Autodesk Inventor part; units mm, degrees
(part 2 of 2)
  line L280 (-42.5388, -23.0761) -> (-41.4675, -19.9061)
  line L281 (-41.4675, -19.9061) -> (-40.5993, -19.9061)
  line L282 (-40.5993, -19.9061) -> (-39.528, -23.0761)
  line L283 (-39.528, -23.0761) -> (-40.3475, -23.0761)
  line L284 (-40.3475, -23.0761) -> (-40.5453, -22.4288)
  line L285 (-40.5453, -22.4288) -> (-41.542, -22.4288)
  line L286 (-41.542, -22.4288) -> (-41.7424, -23.0761)
  line L287 (-41.7424, -23.0761) -> (-42.5388, -23.0761)
  line L288 (-40.72, -21.8533) -> (-41.0437, -20.8052)
  line L289 (-41.0437, -20.8052) -> (-41.3699, -21.8533)
  line L290 (-41.3699, -21.8533) -> (-40.72, -21.8533)
  line L291 (-36.4968, -23.0761) -> (-37.2623, -23.0761)
  line L292 (-37.2623, -23.0761) -> (-38.4851, -20.8669)
  line L293 (-38.4851, -20.8669) -> (-38.4851, -23.0761)
  line L294 (-38.4851, -23.0761) -> (-39.2121, -23.0761)
  line L295 (-39.2121, -23.0761) -> (-39.2121, -19.9061)
  line L296 (-39.2121, -19.9061) -> (-38.2359, -19.9061)
  line L297 (-38.2359, -19.9061) -> (-37.2237, -21.7223)
  line L298 (-37.2237, -21.7223) -> (-37.2237, -19.9061)
  line L299 (-37.2237, -19.9061) -> (-36.4968, -19.9061)
  line L300 (-36.4968, -19.9061) -> (-36.4968, -23.0761)
  line L301 (-50.6873, -28.2954) -> (-50.6873, -25.7291)
  line L302 (-50.6873, -25.7291) -> (-51.6249, -25.7291)
  line L303 (-51.6249, -25.7291) -> (-51.6249, -25.1254)
  line L304 (-51.6249, -25.1254) -> (-48.9533, -25.1254)
  line L305 (-48.9533, -25.1254) -> (-48.9533, -25.7291)
  line L306 (-48.9533, -25.7291) -> (-49.8909, -25.7291)
  line L307 (-49.8909, -25.7291) -> (-49.8909, -28.2954)
  line L308 (-49.8909, -28.2954) -> (-50.6873, -28.2954)
  line L309 (-48.9687, -28.2954) -> (-47.8974, -25.1254)
  line L310 (-47.8974, -25.1254) -> (-47.0292, -25.1254)
  line L311 (-47.0292, -25.1254) -> (-45.9579, -28.2954)
  line L312 (-45.9579, -28.2954) -> (-46.7774, -28.2954)
  line L313 (-46.7774, -28.2954) -> (-46.9752, -27.6481)
  line L314 (-46.9752, -27.6481) -> (-47.9719, -27.6481)
  line L315 (-47.9719, -27.6481) -> (-48.1723, -28.2954)
  line L316 (-48.1723, -28.2954) -> (-48.9687, -28.2954)
  line L317 (-47.1499, -27.0727) -> (-47.4736, -26.0246)
  line L318 (-47.4736, -26.0246) -> (-47.7998, -27.0727)
  line L319 (-47.7998, -27.0727) -> (-47.1499, -27.0727)
  line L320 (-42.7134, -28.2954) -> (-43.6819, -28.2954)
  line L321 (-43.6819, -28.2954) -> (-44.563, -27.1317)
  line L322 (-44.563, -27.1317) -> (-44.8508, -27.1317)
  line L323 (-44.8508, -27.1317) -> (-44.8508, -28.2954)
  line L324 (-44.8508, -28.2954) -> (-45.642, -28.2954)
  line L325 (-45.642, -28.2954) -> (-45.642, -25.1254)
  line L326 (-45.642, -25.1254) -> (-44.3678, -25.1254)
  spline S229 degree 2 poles (-44.3678, -25.1254) (-44.1032, -25.1254) (-43.7127, -25.1922) (-43.5458, -25.295) knots 0 0 0 1 2 2 2
  spline S230 degree 2 poles (-43.5458, -25.295) (-43.3762, -25.4029) (-43.1758, -25.7394) (-43.1758, -25.9963) knots 0 0 0 1 2 2 2
  spline S231 degree 2 poles (-43.1758, -25.9963) (-43.1758, -26.3585) (-43.5047, -26.8132) (-43.7795, -26.9468) knots 0 0 0 1 2 2 2
  line L327 (-43.7795, -26.9468) -> (-42.7134, -28.2954)
  spline S232 degree 2 poles (-43.9927, -26.0965) (-43.9927, -25.9757) (-44.0852, -25.8036) (-44.1906, -25.7574) knots 0 0 0 1 2 2 2
  spline S233 degree 2 poles (-44.1906, -25.7574) (-44.265, -25.7266) (-44.4474, -25.7086) (-44.5836, -25.7086) knots 0 0 0 1 2 2 2
  line L328 (-44.5836, -25.7086) -> (-44.8508, -25.7086)
  line L329 (-44.8508, -25.7086) -> (-44.8508, -26.5615)
  line L330 (-44.8508, -26.5615) -> (-44.6221, -26.5615)
  spline S234 degree 2 poles (-44.6221, -26.5615) (-44.4577, -26.5615) (-44.2239, -26.5203) (-44.1443, -26.4561) knots 0 0 0 1 2 2 2
  spline S235 degree 2 poles (-44.1443, -26.4561) (-44.0672, -26.3945) (-43.9927, -26.2301) (-43.9927, -26.0965) knots 0 0 0 1 2 2 2
  line L331 (-39.8312, -25.1254) -> (-40.9204, -28.2954)
  line L332 (-40.9204, -28.2954) -> (-41.7501, -28.2954)
  line L333 (-41.7501, -28.2954) -> (-42.8393, -25.1254)
  line L334 (-42.8393, -25.1254) -> (-42.0147, -25.1254)
  line L335 (-42.0147, -25.1254) -> (-41.3237, -27.2756)
  line L336 (-41.3237, -27.2756) -> (-40.6352, -25.1254)
  line L337 (-40.6352, -25.1254) -> (-39.8312, -25.1254)
  line L338 (-37.9584, -28.2954) -> (-39.6642, -28.2954)
  line L339 (-39.6642, -28.2954) -> (-39.6642, -27.7431)
  line L340 (-39.6642, -27.7431) -> (-39.2095, -27.7431)
  line L341 (-39.2095, -27.7431) -> (-39.2095, -25.6778)
  line L342 (-39.2095, -25.6778) -> (-39.6642, -25.6778)
  line L343 (-39.6642, -25.6778) -> (-39.6642, -25.1254)
  line L344 (-39.6642, -25.1254) -> (-37.9584, -25.1254)
  line L345 (-37.9584, -25.1254) -> (-37.9584, -25.6778)
  line L346 (-37.9584, -25.6778) -> (-38.4131, -25.6778)
  line L347 (-38.4131, -25.6778) -> (-38.4131, -27.7431)
  line L348 (-38.4131, -27.7431) -> (-37.9584, -27.7431)
  line L349 (-37.9584, -27.7431) -> (-37.9584, -28.2954)
  line L350 (-36.8204, -28.2954) -> (-36.8204, -25.7291)
  line L351 (-36.8204, -25.7291) -> (-37.7581, -25.7291)
  line L352 (-37.7581, -25.7291) -> (-37.7581, -25.1254)
  line L353 (-37.7581, -25.1254) -> (-35.0864, -25.1254)
  line L354 (-35.0864, -25.1254) -> (-35.0864, -25.7291)
  line L355 (-35.0864, -25.7291) -> (-36.0241, -25.7291)
  line L356 (-36.0241, -25.7291) -> (-36.0241, -28.2954)
  line L357 (-36.0241, -28.2954) -> (-36.8204, -28.2954)
  spline S236 degree 2 poles (-47.7587, -32.1199) (-47.7587, -32.8828) (-48.8377, -33.9618) (-49.6006, -33.9618) knots 0 0 0 1 2 2 2
  spline S237 degree 2 poles (-49.6006, -33.9618) (-50.3636, -33.9618) (-51.4425, -32.8828) (-51.4425, -32.1199) knots 0 0 0 1 2 2 2
  spline S238 degree 2 poles (-51.4425, -32.1199) (-51.4425, -31.3569) (-50.3636, -30.278) (-49.6006, -30.278) knots 0 0 0 1 2 2 2
  spline S239 degree 2 poles (-49.6006, -30.278) (-48.8377, -30.278) (-47.7587, -31.3569) (-47.7587, -32.1199) knots 0 0 0 1 2 2 2
  spline S240 degree 2 poles (-48.1646, -32.1199) (-48.1646, -31.5265) (-49.0072, -30.6736) (-49.6006, -30.6736) knots 0 0 0 1 2 2 2
  spline S241 degree 2 poles (-49.6006, -30.6736) (-50.194, -30.6736) (-51.0366, -31.5265) (-51.0366, -32.1199) knots 0 0 0 1 2 2 2
  spline S242 degree 2 poles (-51.0366, -32.1199) (-51.0366, -32.7133) (-50.194, -33.5661) (-49.6006, -33.5661) knots 0 0 0 1 2 2 2
  spline S243 degree 2 poles (-49.6006, -33.5661) (-49.0072, -33.5661) (-48.1646, -32.7133) (-48.1646, -32.1199) knots 0 0 0 1 2 2 2
  spline S244 degree 2 poles (-48.925, -32.9239) (-48.9815, -32.9496) (-49.1023, -33.0036) (-49.187, -33.0267) knots 0 0 0 1 2 2 2
  spline S245 degree 2 poles (-49.187, -33.0267) (-49.2744, -33.0524) (-49.4105, -33.0781) (-49.5158, -33.0781) knots 0 0 0 1 2 2 2
  spline S246 degree 2 poles (-49.5158, -33.0781) (-49.7136, -33.0781) (-50.0707, -32.9599) (-50.2017, -32.8392) knots 0 0 0 1 2 2 2
  spline S247 degree 2 poles (-50.2017, -32.8392) (-50.3353, -32.7158) (-50.4894, -32.3588) (-50.4894, -32.1096) knots 0 0 0 1 2 2 2
  spline S248 degree 2 poles (-50.4894, -32.1096) (-50.4894, -31.8733) (-50.3379, -31.5136) (-50.2043, -31.3877) knots 0 0 0 1 2 2 2
  spline S249 degree 2 poles (-50.2043, -31.3877) (-50.0733, -31.2644) (-49.7136, -31.1334) (-49.5158, -31.1334) knots 0 0 0 1 2 2 2
  spline S250 degree 2 poles (-49.5158, -31.1334) (-49.354, -31.1334) (-49.0534, -31.2208) (-48.925, -31.285) knots 0 0 0 1 2 2 2
  line L358 (-48.925, -31.285) -> (-48.925, -31.7191)
  line L359 (-48.925, -31.7191) -> (-48.9687, -31.7191)
  spline S251 degree 2 poles (-48.9687, -31.7191) (-49.0098, -31.6883) (-49.1048, -31.6215) (-49.1819, -31.583) knots 0 0 0 1 2 2 2
  spline S252 degree 2 poles (-49.1819, -31.583) (-49.2487, -31.5496) (-49.4182, -31.5033) (-49.5056, -31.5033) knots 0 0 0 1 2 2 2
  spline S253 degree 2 poles (-49.5056, -31.5033) (-49.7316, -31.5033) (-49.9757, -31.8116) (-49.9757, -32.1096) knots 0 0 0 1 2 2 2
  spline S254 degree 2 poles (-49.9757, -32.1096) (-49.9757, -32.3999) (-49.7265, -32.7081) (-49.5056, -32.7081) knots 0 0 0 1 2 2 2
  spline S255 degree 2 poles (-49.5056, -32.7081) (-49.4079, -32.7081) (-49.2333, -32.6593) (-49.1716, -32.6259) knots 0 0 0 1 2 2 2
  spline S256 degree 2 poles (-49.1716, -32.6259) (-49.0997, -32.5874) (-49.0021, -32.5206) (-48.9687, -32.4924) knots 0 0 0 1 2 2 2
  line L360 (-48.9687, -32.4924) -> (-48.925, -32.4924)
  line L361 (-48.925, -32.4924) -> (-48.925, -32.9239)
  spline S257 degree 2 poles (-43.7102, -32.1199) (-43.7102, -32.8828) (-44.7891, -33.9618) (-45.5521, -33.9618) knots 0 0 0 1 2 2 2
  spline S258 degree 2 poles (-45.5521, -33.9618) (-46.315, -33.9618) (-47.3939, -32.8828) (-47.3939, -32.1199) knots 0 0 0 1 2 2 2
  spline S259 degree 2 poles (-47.3939, -32.1199) (-47.3939, -31.3569) (-46.315, -30.278) (-45.5521, -30.278) knots 0 0 0 1 2 2 2
  spline S260 degree 2 poles (-45.5521, -30.278) (-44.7891, -30.278) (-43.7102, -31.3569) (-43.7102, -32.1199) knots 0 0 0 1 2 2 2
  spline S261 degree 2 poles (-44.1161, -32.1199) (-44.1161, -31.5265) (-44.9586, -30.6736) (-45.5521, -30.6736) knots 0 0 0 1 2 2 2
  spline S262 degree 2 poles (-45.5521, -30.6736) (-46.1455, -30.6736) (-46.9881, -31.5265) (-46.9881, -32.1199) knots 0 0 0 1 2 2 2
  spline S263 degree 2 poles (-46.9881, -32.1199) (-46.9881, -32.7133) (-46.1455, -33.5661) (-45.5521, -33.5661) knots 0 0 0 1 2 2 2
  spline S264 degree 2 poles (-45.5521, -33.5661) (-44.9586, -33.5661) (-44.1161, -32.7133) (-44.1161, -32.1199) knots 0 0 0 1 2 2 2
  spline S265 degree 2 poles (-44.8764, -32.9239) (-44.933, -32.9496) (-45.0537, -33.0036) (-45.1385, -33.0267) knots 0 0 0 1 2 2 2
  spline S266 degree 2 poles (-45.1385, -33.0267) (-45.2258, -33.0524) (-45.362, -33.0781) (-45.4673, -33.0781) knots 0 0 0 1 2 2 2
  spline S267 degree 2 poles (-45.4673, -33.0781) (-45.6651, -33.0781) (-46.0222, -32.9599) (-46.1532, -32.8392) knots 0 0 0 1 2 2 2
  spline S268 degree 2 poles (-46.1532, -32.8392) (-46.2868, -32.7158) (-46.4409, -32.3588) (-46.4409, -32.1096) knots 0 0 0 1 2 2 2
  spline S269 degree 2 poles (-46.4409, -32.1096) (-46.4409, -31.8733) (-46.2893, -31.5136) (-46.1557, -31.3877) knots 0 0 0 1 2 2 2
  spline S270 degree 2 poles (-46.1557, -31.3877) (-46.0247, -31.2644) (-45.6651, -31.1334) (-45.4673, -31.1334) knots 0 0 0 1 2 2 2
  spline S271 degree 2 poles (-45.4673, -31.1334) (-45.3054, -31.1334) (-45.0049, -31.2208) (-44.8764, -31.285) knots 0 0 0 1 2 2 2
  line L362 (-44.8764, -31.285) -> (-44.8764, -31.7191)
  line L363 (-44.8764, -31.7191) -> (-44.9201, -31.7191)
  spline S272 degree 2 poles (-44.9201, -31.7191) (-44.9612, -31.6883) (-45.0563, -31.6215) (-45.1333, -31.583) knots 0 0 0 1 2 2 2
  spline S273 degree 2 poles (-45.1333, -31.583) (-45.2001, -31.5496) (-45.3697, -31.5033) (-45.457, -31.5033) knots 0 0 0 1 2 2 2
  spline S274 degree 2 poles (-45.457, -31.5033) (-45.6831, -31.5033) (-45.9271, -31.8116) (-45.9271, -32.1096) knots 0 0 0 1 2 2 2
  spline S275 degree 2 poles (-45.9271, -32.1096) (-45.9271, -32.3999) (-45.6779, -32.7081) (-45.457, -32.7081) knots 0 0 0 1 2 2 2
  spline S276 degree 2 poles (-45.457, -32.7081) (-45.3594, -32.7081) (-45.1847, -32.6593) (-45.1231, -32.6259) knots 0 0 0 1 2 2 2
  spline S277 degree 2 poles (-45.1231, -32.6259) (-45.0511, -32.5874) (-44.9535, -32.5206) (-44.9201, -32.4924) knots 0 0 0 1 2 2 2
  line L364 (-44.9201, -32.4924) -> (-44.8764, -32.4924)
  line L365 (-44.8764, -32.4924) -> (-44.8764, -32.9239)
  line L366 (-48.9738, -38.7341) -> (-51.3038, -38.7341)
  line L367 (-51.3038, -38.7341) -> (-51.3038, -38.2177)
  spline S278 degree 2 poles (-51.3038, -38.2177) (-51.0084, -37.9814) (-50.5357, -37.5652) (-50.3584, -37.3777) knots 0 0 0 1 2 2 2
  spline S279 degree 2 poles (-50.3584, -37.3777) (-50.1247, -37.1337) (-49.9166, -36.7612) (-49.9166, -36.566) knots 0 0 0 1 2 2 2
  spline S280 degree 2 poles (-49.9166, -36.566) (-49.9166, -36.345) (-50.1812, -36.1087) (-50.4175, -36.1087) knots 0 0 0 1 2 2 2
  spline S281 degree 2 poles (-50.4175, -36.1087) (-50.5383, -36.1087) (-50.754, -36.1678) (-50.8645, -36.214) knots 0 0 0 1 2 2 2
  spline S282 degree 2 poles (-50.8645, -36.214) (-50.9724, -36.2628) (-51.1265, -36.3656) (-51.1651, -36.3913) knots 0 0 0 1 2 2 2
  line L368 (-51.1651, -36.3913) -> (-51.2267, -36.3913)
  line L369 (-51.2267, -36.3913) -> (-51.2267, -35.7002)
  spline S283 degree 2 poles (-51.2267, -35.7002) (-51.0931, -35.636) (-50.5228, -35.5024) (-50.2582, -35.5024) knots 0 0 0 1 2 2 2
  spline S284 degree 2 poles (-50.2582, -35.5024) (-49.6931, -35.5024) (-49.1125, -36.0059) (-49.1125, -36.4606) knots 0 0 0 1 2 2 2
  spline S285 degree 2 poles (-49.1125, -36.4606) (-49.1125, -36.7406) (-49.3771, -37.2801) (-49.6828, -37.5884) knots 0 0 0 1 2 2 2
  spline S286 degree 2 poles (-49.6828, -37.5884) (-49.8755, -37.7785) (-50.2377, -38.0739) (-50.3173, -38.1355) knots 0 0 0 1 2 2 2
  line L370 (-50.3173, -38.1355) -> (-48.9738, -38.1355)
  line L371 (-48.9738, -38.1355) -> (-48.9738, -38.7341)
  spline S287 degree 2 poles (-46.2379, -37.1491) (-46.2379, -37.5601) (-46.369, -38.1766) (-46.5154, -38.3847) knots 0 0 0 1 2 2 2
  spline S288 degree 2 poles (-46.5154, -38.3847) (-46.6592, -38.5902) (-47.1242, -38.8009) (-47.4582, -38.8009) knots 0 0 0 1 2 2 2
  spline S289 degree 2 poles (-47.4582, -38.8009) (-47.7947, -38.8009) (-48.2571, -38.5902) (-48.4035, -38.3796) knots 0 0 0 1 2 2 2
  spline S290 degree 2 poles (-48.4035, -38.3796) (-48.5499, -38.1715) (-48.681, -37.5601) (-48.681, -37.1491) knots 0 0 0 1 2 2 2
  spline S291 degree 2 poles (-48.681, -37.1491) (-48.681, -36.7278) (-48.5499, -36.1318) (-48.4009, -35.916) knots 0 0 0 1 2 2 2
  spline S292 degree 2 poles (-48.4009, -35.916) (-48.252, -35.7054) (-47.7818, -35.4999) (-47.4582, -35.4999) knots 0 0 0 1 2 2 2
  spline S293 degree 2 poles (-47.4582, -35.4999) (-47.1165, -35.4999) (-46.6592, -35.7157) (-46.5128, -35.9289) knots 0 0 0 1 2 2 2
  spline S294 degree 2 poles (-46.5128, -35.9289) (-46.369, -36.1369) (-46.2379, -36.7509) (-46.2379, -37.1491) knots 0 0 0 1 2 2 2
  spline S295 degree 2 poles (-47.0369, -37.1491) (-47.0369, -36.5608) (-47.2295, -36.0856) (-47.4582, -36.0856) knots 0 0 0 1 2 2 2
  spline S296 degree 2 poles (-47.4582, -36.0856) (-47.6868, -36.0856) (-47.882, -36.5608) (-47.882, -37.1517) knots 0 0 0 1 2 2 2
  spline S297 degree 2 poles (-47.882, -37.1517) (-47.882, -37.7322) (-47.6868, -38.2152) (-47.4582, -38.2152) knots 0 0 0 1 2 2 2
  spline S298 degree 2 poles (-47.4582, -38.2152) (-47.2321, -38.2152) (-47.0369, -37.7322) (-47.0369, -37.1491) knots 0 0 0 1 2 2 2
  line L372 (-43.5612, -38.7341) -> (-45.6548, -38.7341)
  line L373 (-45.6548, -38.7341) -> (-45.6548, -38.1818)
  line L374 (-45.6548, -38.1818) -> (-44.9869, -38.1818)
  line L375 (-44.9869, -38.1818) -> (-44.9869, -36.5043)
  line L376 (-44.9869, -36.5043) -> (-45.6548, -36.5043)
  line L377 (-45.6548, -36.5043) -> (-45.6548, -35.988)
  spline S299 degree 2 poles (-45.6548, -35.988) (-45.5084, -35.988) (-45.2181, -35.9494) (-45.1308, -35.9083) knots 0 0 0 1 2 2 2
  spline S300 degree 2 poles (-45.1308, -35.9083) (-45.0306, -35.8569) (-44.9175, -35.6848) (-44.9073, -35.5564) knots 0 0 0 1 2 2 2
  line L378 (-44.9073, -35.5564) -> (-44.2137, -35.5564)
  line L379 (-44.2137, -35.5564) -> (-44.2137, -38.1818)
  line L380 (-44.2137, -38.1818) -> (-43.5612, -38.1818)
  line L381 (-43.5612, -38.1818) -> (-43.5612, -38.7341)
  spline S301 degree 2 poles (-40.7251, -36.9718) (-40.7251, -37.3752) (-40.9127, -38.0482) (-41.1105, -38.2897) knots 0 0 0 1 2 2 2
  spline S302 degree 2 poles (-41.1105, -38.2897) (-41.316, -38.5337) (-41.9222, -38.7957) (-42.3641, -38.7957) knots 0 0 0 1 2 2 2
  spline S303 degree 2 poles (-42.3641, -38.7957) (-42.5131, -38.7957) (-42.8368, -38.7572) (-42.8907, -38.7418) knots 0 0 0 1 2 2 2
  line L382 (-42.8907, -38.7418) -> (-42.8907, -38.1201)
  line L383 (-42.8907, -38.1201) -> (-42.829, -38.1201)
  spline S304 degree 2 poles (-42.829, -38.1201) (-42.77, -38.151) (-42.549, -38.2177) (-42.3564, -38.2177) knots 0 0 0 1 2 2 2
  spline S305 degree 2 poles (-42.3564, -38.2177) (-42.1997, -38.2177) (-41.9094, -38.1355) (-41.8066, -38.0456) knots 0 0 0 1 2 2 2
  spline S306 degree 2 poles (-41.8066, -38.0456) (-41.6962, -37.9506) (-41.5523, -37.6706) (-41.5266, -37.4599) knots 0 0 0 1 2 2 2
  spline S307 degree 2 poles (-41.5266, -37.4599) (-41.6962, -37.5652) (-41.989, -37.6783) (-42.2074, -37.6783) knots 0 0 0 1 2 2 2
  spline S308 degree 2 poles (-42.2074, -37.6783) (-42.3692, -37.6783) (-42.6698, -37.5909) (-42.7931, -37.4985) knots 0 0 0 1 2 2 2
  spline S309 degree 2 poles (-42.7931, -37.4985) (-42.9575, -37.3726) (-43.1502, -36.9693) (-43.1502, -36.6507) knots 0 0 0 1 2 2 2
  spline S310 degree 2 poles (-43.1502, -36.6507) (-43.1502, -36.4015) (-42.9806, -35.9828) (-42.8265, -35.8287) knots 0 0 0 1 2 2 2
  spline S311 degree 2 poles (-42.8265, -35.8287) (-42.6723, -35.6746) (-42.2254, -35.4999) (-41.9505, -35.4999) knots 0 0 0 1 2 2 2
  spline S312 degree 2 poles (-41.9505, -35.4999) (-41.673, -35.4999) (-41.244, -35.654) (-41.0899, -35.8158) knots 0 0 0 1 2 2 2
  spline S313 degree 2 poles (-41.0899, -35.8158) (-40.9101, -35.9957) (-40.7251, -36.566) (-40.7251, -36.9718) knots 0 0 0 1 2 2 2
  spline S314 degree 2 poles (-41.5138, -36.8537) (-41.5138, -36.5942) (-41.6011, -36.2603) (-41.6808, -36.1678) knots 0 0 0 1 2 2 2
  spline S315 degree 2 poles (-41.6808, -36.1678) (-41.7347, -36.0984) (-41.8734, -36.0393) (-41.9531, -36.0393) knots 0 0 0 1 2 2 2
  spline S316 degree 2 poles (-41.9531, -36.0393) (-42.025, -36.0393) (-42.1586, -36.0958) (-42.2202, -36.1678) knots 0 0 0 1 2 2 2
  spline S317 degree 2 poles (-42.2202, -36.1678) (-42.2742, -36.2294) (-42.3512, -36.4683) (-42.3512, -36.6096) knots 0 0 0 1 2 2 2
  spline S318 degree 2 poles (-42.3512, -36.6096) (-42.3512, -36.7638) (-42.2716, -36.9616) (-42.2048, -37.0206) knots 0 0 0 1 2 2 2
  spline S319 degree 2 poles (-42.2048, -37.0206) (-42.1354, -37.0797) (-41.9633, -37.126) (-41.8554, -37.126) knots 0 0 0 1 2 2 2
  spline S320 degree 2 poles (-41.8554, -37.126) (-41.7655, -37.126) (-41.578, -37.0772) (-41.5189, -37.0515) knots 0 0 0 1 2 2 2
  spline S321 degree 2 poles (-41.5189, -37.0515) (-41.5189, -37.0284) (-41.5138, -36.941) (-41.5138, -36.8537) knots 0 0 0 1 2 2 2
  point P0 (-25, -7.1676)
  point P1 (-34.9687, -21)
  point P2 (-35, -21)
  point P3 (-35, -22)
  point P4 (-3, -22)
  point P5 (-3, -21)
  point P6 (-3.0313, -21)
  point P7 (-19, -6)
  point P8 (-25, -6)
  dimension "d9" = 3.5
  dimension "d10" = 3.5
  dimension "d11" = 3.5
  dimension "d12" = 3.5
  dimension "d13" = 4
  dimension "d14" = 4
  constraints: 64 end point, 12 parallel, 10 point on line, 7 horizontal, 5 centre point, 5 coincident, 5 perpendicular, 2 collinear, 1 midpoint, 1 vertical, 2 other
  measures "d9" diameter of A0
  measures "d10" diameter of A1
  measures "d11" diameter of A2
  measures "d12" diameter of A3
  measures "d13" distance of L28.end L29.end
  measures "d14" distance of L28.start L30.end
extrude "Extrusion4" cut sketch "Sketch4" against normal mid plane 50 contours L97 L98 L99 L9 | L9 L99 L100 L101 L96 L97 | L40 L26 A2 | A2 L38 L40 | A2 L25 L38 | L26 L25 A2 | S48 S49 L9 S50 S51 S52 S53 | L9 S53 S54 S55 S56 S57 S50 S49 S46 S47 S48 | A4 L41 L17 | L17 L9 A4 | L34 L36 A1 | A1 L26 L34 | L41 A4 L9 L17 | L25 L9 A4 | A1 L27 L26 | A4 L9 L27 | L36 L27 A1 | L17 A4 L9 | L9 A4 L17 | L129 L120 L121 L41 | L41 L121 L9 L126 L127 L129 | A3 L25 L24 | L24 L31 A3 | L33 L24 A0 | A0 L29 L33 | L31 L30 A3 | S60 S61 L102 L103 S62 S63 S64 S65 L9 | L9 S65 S66 S67 L104 L105 L106 L107 L108 S58 S59 S60 | L9 L127 L128 L129 | A3 L30 L25 | A0 L24 L27 | L27 L29 A0 | L122 L123 L124 L9 | L121 L122 L9 L124 L125 L126 | L109 L110 L111 L9 L117 L118 | L9 L118 L119 L117 L111 L112 L113 L114 L115 L116 L109 | L42 L43 L44 L45 L46 L47 L48 L49 L50 L51 L52 L53 | L54 L55 L56 L57 L58 L59 L60 L61 L62 L63 L64 L65 | S0 L66 L67 S1 S2 S3 S4 S5 S6 S7 S8 L68 L69 S9 S10 S11 S12 S13 S14 S15 | S16 L70 L71 S17 S18 S19 S20 S21 S22 S23 S24 L72 L73 S25 S26 S27 S28 S29 S30 S31 | L74 L75 L76 L77 L78 L79 L80 L81 | L82 L83 L84 L85 L86 L87 L88 L89 L90 L91 | S32 S33 S34 S35 L92 L93 S36 S37 S38 S39 S40 S41 S42 S43 L94 L95 S44 S45 | L130 L131 L132 L133 L134 L135 L136 L137 | L138 L139 L140 L141 L142 L143 L144 L145 | L149 L150 L151 L152 L153 L154 L155 S68 S69 S70 L156 | L160 L161 L162 L163 L164 L165 L166 | L167 L168 L169 L170 L171 L172 L173 L174 L175 L176 L177 L178 | L179 L180 L181 L182 L183 L184 L185 L186 | S75 S76 S77 S78 | S83 S84 S85 S86 S87 S88 S89 L187 L188 S90 S91 S92 S93 S94 S95 L189 L190 | S96 S97 S98 S99 | S104 S105 S106 S107 S108 S109 S110 L191 L192 S111 S112 S113 S114 S115 S116 L193 L194 | L195 L196 S117 S118 S119 S120 S121 L197 L198 S122 S123 S124 S125 L199 L200 | S126 S127 S128 S129 S130 S131 S132 S133 | L201 L202 L203 L204 L205 L206 S138 S139 L207 L208 L209 L210 | S140 S141 S142 L211 L212 S143 S144 S145 S146 S147 S148 S149 S150 S151 S152
extrude "Extrusion7" cut sketch "Sketch4" against normal blind 10 contours L97 L98 L99 L9 | L9 L99 L100 L101 L96 L97 | S48 S49 L9 S50 S51 S52 S53 | L9 S53 S54 S55 S56 S57 S50 S49 S46 S47 S48 | L129 L120 L121 L41 | L41 L121 L9 L126 L127 L129 | S60 S61 L102 L103 S62 S63 S64 S65 L9 | L9 S65 S66 S67 L104 L105 L106 L107 L108 S58 S59 S60 | L9 L127 L128 L129 | L122 L123 L124 L9 | L121 L122 L9 L124 L125 L126 | L109 L110 L111 L9 L117 L118 | L9 L118 L119 L117 L111 L112 L113 L114 L115 L116 L109 | L42 L43 L44 L45 L46 L47 L48 L49 L50 L51 L52 L53 | L54 L55 L56 L57 L58 L59 L60 L61 L62 L63 L64 L65 | S0 L66 L67 S1 S2 S3 S4 S5 S6 S7 S8 L68 L69 S9 S10 S11 S12 S13 S14 S15 | S16 L70 L71 S17 S18 S19 S20 S21 S22 S23 S24 L72 L73 S25 S26 S27 S28 S29 S30 S31 | L74 L75 L76 L77 L78 L79 L80 L81 | L82 L83 L84 L85 L86 L87 L88 L89 L90 L91 | S32 S33 S34 S35 L92 L93 S36 S37 S38 S39 S40 S41 S42 S43 L94 L95 S44 S45 | L130 L131 L132 L133 L134 L135 L136 L137 | L138 L139 L140 L141 L142 L143 L144 L145 | L149 L150 L151 L152 L153 L154 L155 S68 S69 S70 L156 | L160 L161 L162 L163 L164 L165 L166 | L167 L168 L169 L170 L171 L172 L173 L174 L175 L176 L177 L178 | L179 L180 L181 L182 L183 L184 L185 L186 | S75 S76 S77 S78 | S83 S84 S85 S86 S87 S88 S89 L187 L188 S90 S91 S92 S93 S94 S95 L189 L190 | S96 S97 S98 S99 | S104 S105 S106 S107 S108 S109 S110 L191 L192 S111 S112 S113 S114 S115 S116 L193 L194 | L195 L196 S117 S118 S119 S120 S121 L197 L198 S122 S123 S124 S125 L199 L200 | S126 S127 S128 S129 S130 S131 S132 S133 | L201 L202 L203 L204 L205 L206 S138 S139 L207 L208 L209 L210 | S140 S141 S142 L211 L212 S143 S144 S145 S146 S147 S148 S149 S150 S151 S152
body "Solid1"
